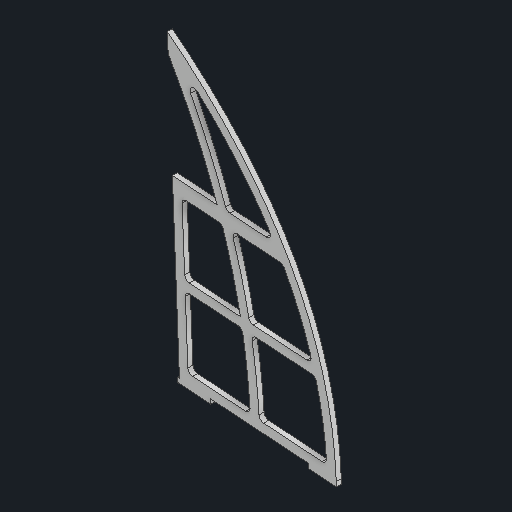
# Autodesk Inventor part: sponson_spanner_side
Saved by Autodesk Inventor 2023 (Build 270158030, 158C)
## iProperties
Created: 2022-03-22
Part Number: sponson_spanner_side
Material: Generic
Document SubType Name: Modeling
Designer: kardo
Density: 1 g/cm^3
Appearance: Default
Author: kardo
Autodesk Inventor part; units mm, degrees
ref_plane "YZ Plane" through (0, 0, 0) normal (1, 0, 0) x (0, 1, 0)
ref_plane "XZ Plane" through (0, 0, 0) normal (0, 1, 0) x (-1, 0, 0)
ref_plane "XY Plane" through (0, 0, 0) normal (0, 0, 1) x (1, 0, 0)
derived "surface_body.ipt"
sketch "sk_rail_sponson_side" plane through (81.12, 255, 36.448) normal (0.06099, 0.0391867, -0.9973689) x (0.2816917, -0.9592867, -0.0204648)
  line L0 (265.8225, 0) -> (150.2798, -33.9898)
  spline S0 degree 2 poles (150.2798, -33.9898) (71.6973, -57.1068) (0, 0) knots 0 0 0 1 1 1
  point P0 (222.5132, 151.5365)
ref_plane "plane_tunnel_right" through (81.12, 0, 0) normal (1, 0, 0) x (0, 1, 0)
ref_plane "plane_sponson_side" through (81.12, 255, 36.448) normal (0.06099, 0.0391867, -0.9973689) x (0.2816917, -0.9592867, -0.0204648)
sketch "sk_rail_sponson_tunnel" plane through (81.12, 0, 0) normal (1, 0, 0) x (0, 1, 0)
  line L0 (0, 0) -> (122.4, 9.6331)
  line L1 (111.1171, 152.996) -> (142.2856, -243.0375) construction
  spline S0 degree 2 poles (122.4, 9.6331) (190.08, 14.9596) (255, 36.448) knots 0 0 0 1 1 1
sketch "sk_rail_sponson_bottom" plane through (126.048, 0, 0) normal (0.341579, -0.07374, 0.9369558) x (-0.1718217, 0.9752166, 0.139391)
  line L0 (120.7093, -22.4461) -> (0, 0)
  line L1 (389.6045, -72.4475) -> (-475.366, 88.395) construction
  line L2 (163.4334, 207.3137) -> (92.7222, -172.9535) construction
  spline S0 degree 2 poles (120.7093, -22.4461) (192.8116, -35.8536) (261.4804, 0) knots 0 0 0 1 1 1
  point P0 (21.6578, 116.4701)
sketch "sk_rail_top_tunnel" plane through (81.12, 0, 0) normal (1, 0, 0) x (0, 1, 0)
  line L0 (255, 107.6209) -> (255, -224.5198) construction
  line L1 (0, 107.6209) -> (0, -224.5198) construction
  line L2 (-345, 107.6209) -> (-345, -224.5198) construction
  line L3 (-345, 0) -> (0, 0) construction
  line L4 (-172.5, 48.8998) -> (-172.5, 0) construction
  line L5 (0, 52.89) -> (37.026, 52.89) construction
  line L6 (37.026, 52.89) -> (80.784, 47.0555) construction
  line L7 (80.784, 47.0555) -> (112.2, 37.536) construction
  line L8 (112.2, 107.6209) -> (112.2, -224.5198) construction
  line L9 (0, 52.89) -> (255, 52.89) construction
  line L10 (-469.9275, 0) -> (379.2584, 0) construction
  spline S0 degree 3 poles (0, 52.89) (92.8353, 52.89) (195.0311, 49.5089) (255, 36.448) knots 0 0 0 0 1 1 1 1
  spline S1 degree 3 poles (0, 52.89) (37.026, 52.89) (80.784, 47.0555) (112.2, 37.536) knots 1 1 1 1 2 2 2 2
  spline S2 degree 4 poles (-345, 37.3935) (-258.8686, 45.1235) (-172.5923, 49.7074) (-86.3167, 52.89) (0, 52.89) knots 0 0 0 0 0 1 1 1 1 1
  point P0 (153, 48.7795)
  point P1 (112.2, 28.832)
  point P2 (-230.0001, 45.8224)
  point P3 (-114.9999, 50.9907)
sketch "sk_section_sponson_break" plane through (0, 122.4, 9.6331) normal (0, 0.9969173, 0.0784591) x (-1, 0, 0)
  line L0 (-268.0445, -51.607) -> (63.6955, 68.9601) construction
  line L1 (-81.12, -266.2886) -> (-81.12, 157.0776) construction
  arc A0 (-81.12, 41.081) -> (-156, 26.184) centre (-72.7535, -196.6143) ccw construction
  arc A1 (-54.6, 54.2323) -> (-156, 30.9124) centre (-53.2835, -183.6066) ccw construction
  spline S0 degree 2 poles (-54.6, 54.2323) (-107.2974, 54.2323) (-156, 30.9124) knots 0 0 0 1 1 1
  spline S1 degree 2 poles (-156, 26.184) (-120.0091, 39.6317) (-81.12, 41.081) knots 0 0 0 1 1 1
  point P0 (0, 0)
ref_plane "plane_sponson_break" through (0, 122.4, 9.6331) normal (0, 0.9969173, 0.0784591) x (-1, 0, 0)
derived "parameters_frame.ipt"
derived "stencil_frame.ipt"
sketch "sk_joint_locations" plane through (81.12, 0, 0) normal (1, 0, 0) x (0, 1, 0)
  line L0 (0, 0) -> (122.4, 9.6331) construction
  line L1 (36.465, 28.832) -> (112.2, 28.832) construction
  arc A0 (36.465, 28.832) -> (11.22, 28.376) centre (36.465, -670.197) ccw construction
  line L2 (-241.5001, 19.2432) -> (11.22, 28.376) construction
  line L3 (-345, 16.32) -> (-262.2001, 18.586) construction
  arc A1 (-262.2001, 18.586) -> (-241.5001, 19.2432) centre (-326.8578, 2381.2399) ccw construction
  line L4 (-122.4795, 3121.122) -> (270.8781, -1876.9598) construction
  line L5 (-230.0001, 3089.1136) -> (-230.0001, -1866.0023) construction
  line L6 (-114.9999, 3089.1136) -> (-114.9999, -1866.0023) construction
  line L7 (-345, 3089.1136) -> (-345, -1866.0023) construction
  line L8 (0, 3089.1136) -> (0, -1866.0023) construction
  line L9 (529.622, 47.2379) -> (-602.608, 2.7525) construction
  line L10 (-673.1615, -36.5999) -> (647.9226, 67.3717) construction
  line L11 (193.439, 30.0262) -> (193.1249, 38.02) construction
  line L12 (201.1327, 36.2333) -> (201.7624, 28.2333) construction
  line L13 (0, 14.144) -> (121.9006, 15.9783) construction
  line L14 (-230.0001, 45.8224) -> (-230.0001, 19.6588) construction
  line L15 (-345, 37.3935) -> (-345, 16.32) construction
  line L16 (-114.9999, 50.9907) -> (-114.9999, 23.8147) construction
  line L17 (0, 52.89) -> (0, 27.9705) construction
  line L18 (119.1768, 50.5875) -> (119.7216, 43.6656) construction
  line L19 (120.2663, 36.7438) -> (119.7216, 43.6656) construction
  line L20 (120.2663, 36.7438) -> (120.8111, 29.822) construction
  line L21 (120.8111, 29.822) -> (121.3559, 22.9001) construction
  line L22 (121.3559, 22.9001) -> (121.9006, 15.9783) construction
  line L23 (0, 14.144) -> (0, 0) construction
  line L24 (112.2, 37.536) -> (112.2, 28.832) construction
  line L25 (112.2, 35.548) -> (112.2, 30.82) construction
  spline S0 degree 4 poles (-345, 37.3935) (-258.8686, 45.1235) (-172.5923, 49.7074) (-86.3167, 52.89) (0, 52.89) knots 0 0 0 0 0 1 1 1 1 1
  spline S1 degree 3 poles (0, 52.89) (92.8353, 52.89) (195.0311, 49.5089) (255, 36.448) knots 0 0 0 0 1 1 1 1
  spline S2 degree 2 poles (122.4, 9.6331) (190.08, 14.9596) (255, 36.448) knots 0 0 0 1 1 1
  point P0 (-122.4795, 3121.122)
  point P1 (270.8781, -1876.9598)
  point P2 (193.282, 34.0231)
  point P3 (201.4475, 32.2333)
  point P4 (134.9575, 11.3411)
  point P5 (-345, 26.8568)
  point P6 (-230.0001, 32.7406)
  point P7 (-114.9999, 37.4027)
  point P8 (0, 40.4303)
  point P9 (112.2, 33.184)
sketch "sk_spanner_joints_locations" plane through (0, 122.4, 9.6331) normal (0, 0.9969173, 0.0784591) x (-1, 0, 0)
  line L0 (328.7115, -3.4565) -> (-466.2934, 45.1587) construction
  line L1 (-867.9776, -269.6459) -> (1175.5999, 473.0692) construction
  line L2 (-83.4141, 21.7453) -> (-82.5545, 15.8072) construction
  line L3 (-83.4141, 21.7453) -> (-68.6928, 20.8451) construction
  line L4 (-82.5545, 15.8072) -> (-68.6928, 20.8451) construction
  point P0 (0, 0)
  point P1 (-126.048, 0)
  point P2 (-156, 26.184)
  point P3 (-141.4828, 25.2963)
  point P4 (-97.9313, 22.6331)
  point P5 (-93.4279, 11.8554)
  point P6 (-115.1746, 3.9518)
ref_plane "plane_stringer_outer" through (84.12, 0, 0) normal (1, 0, 0) x (0, 1, 0)
sketch "sk_corner_offset" plane through (0, 122.4, 9.6331) normal (0, 0.9969173, 0.0784591) x (-1, 0, 0)
  spline S0 degree 2 poles (-156, 26.184) (-120.0091, 39.6317) (-81.12, 41.081) knots 0 0 0 1 1 1 construction
  line L0 (-156, 26.184) -> (-126.048, 0) construction
  line L1 (-153.6888, 25.7575) -> (-125.2582, 0.9035) construction
  line L2 (-125.2582, 0.9035) -> (-126.048, 0) construction
  spline S1 degree 5 poles (-153.6888, 25.7575) (-139.7296, 30.8396) (-125.3756, 34.8381) (-110.7246, 37.6698) (-95.9206, 39.3284) (-81.0753, 39.8819) knots 0 0 0 0 0 0 1 1 1 1 1 1 construction
  point P0 (0, 0)
  dimension "d9" = 1.2
  dimension "d10" = 1.2
  constraints: 6 end point, 1 coincident, 1 parallel, 1 perpendicular, 3 other
  measures "d10" distance between parallel lines of L1 L0
sketch "sk_tip_offset" plane through (81.12, 0, 0) normal (1, 0, 0) x (0, 1, 0)
  spline S0 degree 3 poles (0, 52.89) (92.8353, 52.89) (195.0311, 49.5089) (255, 36.448) knots 0 0 0 0 1 1 1 1 construction
  spline S1 degree 2 poles (122.4, 9.6331) (190.08, 14.9596) (255, 36.448) knots 0 0 0 1 1 1 construction
  spline S2 degree 5 poles (0, 51.69) (14.1108, 51.69) (28.2217, 51.6249) (42.3321, 51.4877) (70.2924, 51.0558) (98.2445, 50.2552) (112.0882, 49.7555) (138.5614, 48.5709) (165.0044, 46.8436) (177.6143, 45.8726) (199.7992, 43.8515) (221.9015, 41.0762) (231.4314, 39.7015) (240.9325, 38.1149) (250.3665, 36.1966) knots 0 0 0 0 0 0 0.280891 0.280891 0.280891 0.556633 0.556633 0.556633 0.808364 0.808364 0.808364 1 1 1 1 1 1 construction
  spline S3 degree 4 poles (122.3058, 10.8294) (154.9158, 13.3957) (187.3327, 18.4882) (219.233, 26.1601) (250.3665, 36.1967) knots 0 0 0 0 0 1 1 1 1 1 construction
  point P0 (0, 0)
  dimension "d7" = 1.2
  dimension "d8" = 1.2
  constraints: 1 coincident, 6 other
sketch "sk_sponson_spanner_side_base" plane through (81.12, 255, 36.448) normal (0.06099, 0.0391867, -0.9973689) x (0.2816917, -0.9592867, -0.0204648)
  spline S0 degree 2 poles (150.2798, -33.9898) (71.6973, -57.1068) (0, 0) knots 0 0 0 1 1 1 construction
  line L0 (129.5894, 35.7262) -> (129.7906, 35.0482)
  line L1 (133.7275, 21.783) -> (146.1417, -20.0466)
  line L2 (146.1417, -20.0466) -> (148.0591, -19.4776)
  line L3 (148.0591, -19.4776) -> (151.5348, -31.1889)
  line L4 (133.7275, 21.783) -> (135.6448, 22.3521)
  line L5 (135.6448, 22.3521) -> (131.5068, 36.2953)
  line L6 (131.5068, 36.2953) -> (129.5894, 35.7262)
  line L7 (748.8189, 217.151) -> (-250.2454, -76.7489) projected
  line L8 (151.5348, -31.1889) -> (149.6053, -31.7565)
  line L9 (265.8225, 0) -> (150.2798, -33.9898) construction
  spline S1 degree 2 poles (4.45, 1.3135) (73.6482, -54.1012) (149.6053, -31.7565) knots 0 0 0 1 1 1
  point P0 (222.5132, 151.5365)
  point P1 (59.2549, 17.4313)
  point P2 (99.6986, 28.3676)
  point P3 (2.9047, -2.2785)
  point P4 (7.3485, -0.9712)
  dimension "d3" = 2
  constraints: 16 end point, 4 parallel, 2 collinear, 2 perpendicular, 1 point on line, 3 other
  measures "d3" distance between parallel lines of L5 L1
extrude "thicken" add sketch "sk_sponson_spanner_side_base" along normal blind 2
sketch "sk_cut_weight" plane through (81.12, 255, 36.448) normal (0.06099, 0.0391867, -0.9973689) x (0.2816917, -0.9592867, -0.0204648)
  line L0 (129.5894, 35.7262) -> (129.7906, 35.0482) construction
  line L1 (133.7275, 21.783) -> (146.1417, -20.0466) construction
  spline S0 degree 2 poles (4.45, 1.3135) (73.6482, -54.1012) (149.6053, -31.7565) knots 0 0 0 1 1 1 construction
  line L2 (59.2549, 17.4313) -> (73.2202, -30.0413) construction
  line L3 (65.0694, 11.8394) -> (70.0882, -5.221)
  line L4 (58.1845, 13.9835) -> (63.8017, -5.1115)
  line L5 (58.1845, 13.9835) -> (15.0113, 1.283)
  line L6 (65.0694, 11.8394) -> (127.0913, 30.0847)
  line L7 (127.0913, 30.0847) -> (134.9527, 3.5957)
  line L8 (71.2655, -9.223) -> (77.6976, -31.0881)
  line L9 (64.9886, -9.1462) -> (70.9628, -29.4545)
  line L10 (136.0909, -0.2395) -> (144.6269, -29.0016)
  line L11 (96.0804, 20.962) -> (112.2655, -34.0569) construction
  line L12 (101.1314, -3.2948) -> (94.1617, 20.3976)
  line L13 (97.9991, 21.5265) -> (105.1384, -2.7427)
  line L14 (106.2784, -6.6177) -> (114.3205, -33.9557)
  line L15 (102.2742, -7.1796) -> (110.2017, -34.1277)
  line L16 (748.8189, 217.151) -> (-250.2454, -76.7489) construction
  spline S1 degree 2 poles (139.9346, 0.8682) (75.1843, -18.3484) (7.3485, -0.9712) knots 0 0 0 1 1 1
  spline S2 degree 5 poles (17.1876, -3.3027) (23.8662, -8.0532) (30.7726, -12.4833) (37.9126, -16.5418) (54.0078, -24.4532) (71.0777, -30.0002) (80.5766, -32.2122) (99.2096, -34.7919) (117.9986, -34.142) (127.0117, -33.0812) (135.8998, -31.3422) (144.6269, -29.0016) knots 0 0 0 0 0 0 0.304319 0.304319 0.304319 0.664493 0.664493 0.664493 1 1 1 1 1 1
  spline S3 degree 5 poles (134.9527, 3.5957) (123.125, 0.2917) (111.0925, -2.2784) (98.9049, -4.061) (74.6801, -5.9743) (50.4118, -4.7738) (38.4881, -3.4349) (26.676, -1.397) (15.0113, 1.283) knots 0 0 0 0 0 0 0.50643 0.50643 0.50643 1 1 1 1 1 1
  point P0 (222.5132, 151.5365)
  dimension "d11" = 4
  dimension "d20" = 4
  dimension "d14" = 2
  dimension "d15" = 4
  dimension "d16" = 4
  dimension "d19" = 4
  dimension "d21" = 4
  constraints: 28 end point, 6 collinear, 5 parallel, 3 point on line, 2 midpoint, 2 perpendicular, 28 other
  measures "d14" distance between parallel lines of L2 L4
  measures "d15" distance between parallel lines of L2 L3
  measures "d16" distance between parallel lines of L1 L7
  measures "d19" distance between parallel lines of L13 L12
  measures "d21" distance between parallel lines of L16 L6
extrude "cut_weight" cut sketch "sk_cut_weight" along normal through all both and the other way through all contours L6 L12 S3 L3 | L6 L7 S3 L13 | L4 S3 L5 | S1 L15 S2 L8 | L9 S2 S1 | S1 L10 S2 L14
fillet "rounding" radius 2 18 edges at (88.1735, 124.7075, 30.7575) (119.746, 124.556, 32.6822) (116.8657, 158.9371, 33.8569) (88.1735, 159.0059, 32.1051) (108.2458, 195.2547, 34.7567) (88.1735, 155.009, 31.948) (88.1735, 189.3075, 33.2956) (110.0875, 189.2549, 34.6336) (89.1852, 239.4751, 35.3286) (117.4556, 154.9387, 33.7359) (105.9237, 189.2649, 34.3794) (132.8366, 189.2003, 36.0226) (113.4239, 154.9484, 33.4897) (145.8989, 154.8705, 35.4726) (129.3752, 195.204, 36.0468) (149.6921, 124.4123, 34.5078) (144.9034, 158.8698, 35.5688) (115.753, 124.5751, 32.4388)
equation "\"d9\" = shell_thickness"
equation "\"d10\" = shell_thickness"
equation "\"d7\" = shell_thickness"
equation "\"d8\" = shell_thickness"
equation "\"d3\" = bulkhead_thickness"
equation "\"d5\" = bulkhead_thickness"
equation "\"d11\" = bulkhead_inset"
equation "\"d20\" = bulkhead_inset"
equation "\"d14\" = bulkhead_thickness"
equation "\"d15\" = 2 * bulkhead_thickness"
equation "\"d16\" = bulkhead_inset"
equation "\"d19\" = bulkhead_inset"
equation "\"d21\" = bulkhead_inset"
equation "\"d25\" = 0.5 * bulkhead_inset"
equation "\"d4\" = stringer_thickness"
equation "\"shell_thickness\" = 1.2"
equation "\"bulkhead_thickness\" = 2"
equation "\"bulkhead_inset\" = 4"
equation "\"stringer_thickness\" = 3"
body "Solid1"
